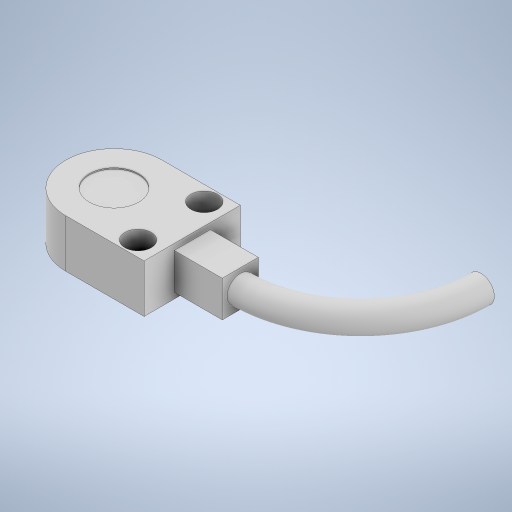
# Autodesk Inventor part: CapacitiveSensor
Saved by Autodesk Inventor 2023 (Build 270158000, 158)
## iProperties
Created: 2023-04-24
Part Number: CapacitiveSensor
Material: Generic
Document SubType Name: Modeling
Designer: Nathann
Density: 1 g/cm^3
Appearance: Default
Author: Nathann
Autodesk Inventor part; units mm, degrees
ref_plane "YZ Plane" through (0, 0, 0) normal (1, 0, 0) x (0, 1, 0)
sketch "Sketch1" plane through (0, 0, 0) normal (0, 1, 0) x (-1, 0, 0)
  circle A0 centre (0, 0) radius 4
  line L0 (0, 4) -> (-6.5, 4)
  line L1 (-6.5, 4) -> (-6.5, -4)
  line L2 (-6.5, -4) -> (0, -4)
  line L3 (0, -4) -> (0, 4)
  circle A1 centre (-4.75, 2.75) radius 1.1
  circle A2 centre (-4.75, -2.75) radius 1.1
  point P0 (-6.5, 0)
  dimension "d0" = 8
  dimension "d1" = 6.5
  dimension "d2" = 5.5
  dimension "d3" = 2.75
  dimension "d4" = 1.75
  dimension "d5" = 1.75
  dimension "d6" = 2.2
  dimension "d7" = 2.2
  constraints: 8 end point, 2 centre point, 2 parallel, 1 coincident, 1 horizontal, 1 midpoint, 1 perpendicular, 3 other
  measures "d1" distance of L1.end L2.end
  measures "d2" distance of A2.centre A1.centre
  measures "d3" vertical distance of A1.centre point (-6.5, 0)
  measures "d4" distance from line of L1 A1.centre
  measures "d5" distance from line of L1 A2.centre
  measures "d6" diameter of A1
  measures "d7" diameter of A2
extrude "Extrusion1" add sketch "Sketch1" along normal blind 4
sketch "Sketch2" plane through (6.5, 0, 4) normal (1, 0, 0) x (0, 0, -1)
  line L0 (2.5, 3.5) -> (5.5, 3.5)
  line L1 (5.5, 3.5) -> (5.5, 0.5)
  line L2 (5.5, 0.5) -> (2.5, 0.5)
  line L3 (2.5, 0.5) -> (2.5, 3.5)
  line L4 (0, 4) -> (8, 4) projected
  line L5 (8, 0) -> (8, 4) projected
  point P0 (4, 0)
  dimension "d10" = 3
  dimension "d11" = 3
  dimension "d12" = 0.5
  dimension "d13" = 5.5
  constraints: 8 end point, 2 parallel, 1 horizontal, 1 perpendicular
  measures "d10" distance of L2.end L0.start
  measures "d11" distance of L0.start L0.end
  measures "d12" distance between parallel lines of L4 L0
  measures "d13" distance between parallel lines of L5 L3
extrude "Extrusion2" add sketch "Sketch2" along normal blind 4
sketch "Sketch3" plane through (0, 4, 0) normal (0, 1, 0) x (1, 0, 0)
  circle A0 centre (0, 0) radius 2.05
  dimension "d16" = 4.1
  constraints: 1 centre point, 1 coincident
  measures "d16" diameter of A0
extrude "Extrusion3" cut sketch "Sketch3" against normal blind 0.1
sketch "Sketch4" plane through (10.5, 0, 4) normal (1, 0, 0) x (0, 0, -1)
  circle A0 centre (4, 2) radius 1.1
  point P0 (4, 0)
  dimension "d19" = 2.2
  constraints: 1 centre point
  measures "d19" diameter of A0
ref_plane "Work Plane2" through (6.5, 0.5, -10) normal (0, 0, 1) x (1, 0, 0)
ref_plane "Work Plane1" through (6.5, 0.5, 0) normal (0, 0, 1) x (1, 0, 0)
sketch "Sketch5" plane through (6.5, 0.5, -10) normal (0, 0, 1) x (1, 0, 0)
  circle A0 centre (14, 1.7321) radius 1.1
  line L0 (4, 0) -> (4, 3) projected
  point P0 (-6.5, -0.5)
  dimension "d23" = 10
  dimension "d24" = 2.2
  constraints: 1 centre point
  measures "d23" distance from line of A0.centre L0
  measures "d24" diameter of A0
ref_plane "Work Plane3" through (6.5, 2, -1.5) normal (0, -1, 0) x (1, 0, 0)
sketch "Sketch6" plane through (6.5, 2, -1.5) normal (0, -1, 0) x (1, 0, 0)
  circle A0 centre (4, -8.5) radius 10
  line L0 (4, 3) -> (4, 0) projected
  point P0 (-6.5, 1.5)
  point P1 (4, 1.5)
  dimension "d25" = 20
  dimension "d26" = 10
  constraints: 1 centre point, 1 midpoint
  measures "d25" diameter of A0
  measures "d26" distance of point (4, 1.5) A0.centre
revolve "Revolution1" add sketch "Sketch4" angle 90 about axis through (10.5, 0.5, -10) along (0, 1, 0)
equation "\"d3\" = 0.5 * d2"
equation "\"d5\" = d4"
equation "\"d6\" = d7"
body "Solid1"
